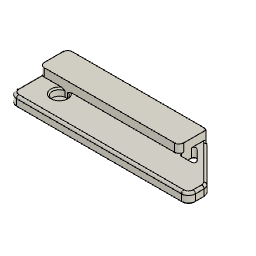
Handle Nameplate (Autodesk Fusion 360 design; units mm, degrees)
Autodesk Fusion 360 part; units mm, degrees
sketch "Sketch1" plane through (0, 0, 0) normal (0, 0, 1) x (1, 0, 0)
  line L0 (0, 0) -> (-60, 0)
  line L1 (-60, 0) -> (-60, 12)
  line L2 (-60, 12) -> (0, 12)
  line L3 (0, 12) -> (0, 0)
  dimension "d1" = 60
  dimension "d2" = 12
  constraint horizontal L0
  constraint vertical L1
  constraint horizontal L2
  constraint vertical L3
  constraint coincident L0.start L3.end
  measures "d1" distance of L0.start L0.end
  measures "d2" distance of L0.start L2.end
extrude "Extrude1" add sketch "Sketch1" along normal blind 7.5
sketch "Sketch2" plane through (0, 0, 0) normal (0, 0, -1) x (1, 0, 0)
  line L0 (-60, -12) -> (0, -12)
  line L1 (0, -12) -> (0, 0)
  line L2 (0, 0) -> (-60, 0)
  line L3 (-60, 0) -> (-60, -12)
  line L4 (-60, 0) -> (-60, 13)
  line L5 (-60, 13) -> (17, 13)
  line L6 (0, -12) -> (17, 5)
  line L7 (17, 5) -> (17, 13)
  dimension "d5" = 25
  dimension "d6" = 17
  dimension "d7" = 45
  constraint coincident L2.end L3.start
  constraint perpendicular L2 L4
  constraint perpendicular L4 L5
  constraint coincident L0.end L1.start
  constraint coincident L5 L7.end
  constraint perpendicular L5 L7
  measures "d5" distance of L0.start L4.end
  measures "d6" horizontal distance of L0.end L6.end
  measures "d7" angle of L1 L6
extrude "Extrude2" add sketch "Sketch2" against normal blind 4 contours L1 L2 L4 L5 L6 L7
sketch "Sketch3" plane through (0, 0, 4) normal (0, 0, 1) x (-1, 0, 0)
  line L0 (-17, 5) -> (0, -12)
  line L1 (0, -12) -> (0, 0)
  line L2 (0, 0) -> (60, 0)
  line L3 (60, 0) -> (60, 13)
  line L4 (60, 13) -> (-17, 13)
  line L5 (-17, 13) -> (-17, 5)
  line L6 (48.535, 0) -> (48.535, 3) construction
  circle A0 centre (48.535, 3) radius 3.05
  dimension "d10" = 11.465
  dimension "d11" = 6.1
  dimension "d12" = 3
  constraint coincident L2 L6.start
  constraint perpendicular L2 L6
  constraint coincident L6.end A0.centre
  measures "d10" distance of L2.end L6.start
  measures "d11" diameter of A0
  measures "d12" distance of L6.start L6.end
extrude "Extrude3" cut sketch "Sketch3" along normal up to surface (3.5 mm away) and the other way blind 3 contours L2 A0 picked at (49.8828, 1.8084)
sketch "Sketch4" plane through (0, 0, 4) normal (0, 0, 1) x (-1, 0, 0)
  arc A0 (49.085, 0) -> (47.985, 0) centre (48.535, 3) ccw
  line L0 (49.085, 0) -> (60, 0)
  line L1 (60, 0) -> (60, 13)
  line L2 (60, 13) -> (-17, 13)
  line L3 (-17, 13) -> (-17, 5)
  line L4 (-17, 5) -> (0, -12)
  line L5 (0, -12) -> (0, 0)
  line L6 (0, 0) -> (47.985, 0)
  line L7 (0, 0) -> (-7.7574, 0)
  line L8 (-7.7574, 0) -> (0, -7.7574)
  dimension "d17" = 3
  constraint coincident L5.end L6.start
  constraint perpendicular L5 L7
  constraint coincident L5 L8.end
  constraint parallel L4 L8
  measures "d17" distance of L4 L8
extrude "Extrude4" cut sketch "Sketch4" against normal through all contours L5 L7 L8
extrude "Extrude5" add 1 faces at (-40, -0.3333, 0) along direction (0, 0, -1) blind 0.4
sketch "Sketch7" plane through (0, 0, -0.4) normal (0, 0, -1) x (1, 0, 0)
  line L0 (7.7574, 0) -> (0, -7.7574)
  line L1 (0, -7.7574) -> (0, 0)
  line L2 (0, 0) -> (7.7574, 0)
  line L3 (-60, -12) -> (0, -12)
  line L4 (0, -12) -> (17, 5)
  line L5 (17, 5) -> (17, 13)
  line L6 (17, 13) -> (-60, 13)
  line L7 (-60, 13) -> (-60, -12)
  line L8 (-30, -12) -> (-30, 13) construction
  line L9 (-55.25, 10.75) -> (-4.75, 10.75)
  line L10 (-4.75, 10.75) -> (-4.75, -9.75)
  line L11 (-4.75, -9.75) -> (-55.25, -9.75)
  line L12 (-55.25, -9.75) -> (-55.25, 10.75)
  line L13 (-4.75, -9.75) -> (-55.25, 10.75) construction
  dimension "d35" = 20.5
  dimension "d36" = 50.5
  constraint midpoint L3 L8.start
  constraint coincident L6 L8.end
  constraint perpendicular L6 L8
  constraint horizontal L9
  constraint vertical L10
  constraint horizontal L11
  constraint vertical L12
  constraint midpoint L8 L13
  measures "d35" distance of L9.start L11.end
  measures "d36" distance of L9.start L9.end
extrude "Extrude6" cut sketch "Sketch7" against normal blind 1 contours L9 L10 L11 L12
fillet "Fillet1" radius 3 3 edges at (17, -13, 2) (17, -5, 2) (-60, -13, 2)
fillet "Fillet2" radius 2 3 edges at (-60, 12, 3.75) (0, 0, 5.75) (-60, 0, 5.75)
fillet "Fillet3" radius 5 2 edges at (0, 12, 2) (0, 12, 5.75)
fillet "Fillet4" radius 1 3 edges at (0, 7.7574, 2) (7.7574, 0, 2) (0, 0, 2)
fillet "Fillet5" radius 1 8 edges at (-60, -4, 4) (-59.1213, -12.1213, 4) (-21.5, -13, 4) (16.1213, -12.1213, 4) (17, -8.1213, 4) (16.7716, -5.0946, 4) (8.7929, 3.2071, 4) (0.7778, 11.109, 4)
chamfer "Chamfer1" distance 0.6 angle 45 16 edges at (-30.0355, 12, -0.4) (-0.1577, 11.6194, -0.4) (8.7929, 3.2071, -0.4) (16.7716, -5.0946, -0.4) (17, -8.1213, -0.4) (16.1213, -12.1213, -0.4) (-21.5, -13, -0.4) (-59.1213, -12.1213, -0.4) (-60, 0, -0.4) (-59.4142, 11.4142, -0.4) (0, 3.1716, -0.4) (0.2929, 0.2929, -0.4) (3.1716, 0, -0.4) (6.267, 0.6173, -0.4) (3.8787, 3.8787, -0.4) (0.6173, 6.267, -0.4)
chamfer "Chamfer2" distance 0.6 angle 45 1 edges at (-48.535, -6.05, 4)
fillet "Fillet6" radius 1 4 edges at (-4.75, -10.75, 0.1) (-55.25, -10.75, 0.1) (-55.25, 9.75, 0.1) (-4.75, 9.75, 0.1)
equation "d10 = ( 22.93 / 2 ) * 1 mm"
